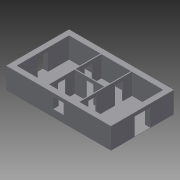
# Autodesk Inventor part: East_Structure
Saved by Autodesk Inventor 2013 SP2 (Build 170200200, 200)
## iProperties
Created: 2014-07-16
Part Number: East_Structure
Material: Generic
Document SubType Name: Modeling
Designer: jmw3
Density: 1 g/cm^3
Author: jmw3
Autodesk Inventor part; units mm, degrees
ref_plane "YZ Plane" through (0, 0, 0) normal (1, 0, 0) x (0, 1, 0)
ref_plane "XZ Plane" through (0, 0, 0) normal (0, 1, 0) x (-1, 0, 0)
ref_plane "XY Plane" through (0, 0, 0) normal (0, 0, 1) x (1, 0, 0)
sketch "Sketch1" plane through (0, 0, 0) normal (0, 1, 0) x (-1, 0, 0)
  line L0 (3657.6, -6096) -> (3657.6, 6096)
  line L1 (-3657.6, 6096) -> (-3657.6, -6096)
  line L2 (-5120.64, 0) -> (5120.64, 0) projected
  line L3 (0, -16303.5007) -> (0, 17151.3473) projected
  line L4 (-3048, 1714.5) -> (-3048, -1714.5)
  line L5 (3048, -5486.4) -> (3048, -1828.8)
  line L6 (3048, -1714.5) -> (3048, 1714.5)
  line L7 (3048, 1828.8) -> (3048, 5486.4)
  line L8 (-3048, -1828.8) -> (-3048, -5486.4)
  line L9 (-3048, 5486.4) -> (-3048, 1828.8)
  line L10 (-3048, 1714.5) -> (-3048, -1714.5)
  line L11 (-2009.775, -1828.8) -> (-2009.775, -1714.5)
  line L12 (-1095.375, -1828.8) -> (-1095.375, -1714.5)
  line L13 (-3048, -1714.5) -> (-2009.775, -1714.5)
  line L14 (-1095.375, -1714.5) -> (-57.15, -1714.5)
  line L15 (-3048, -1828.8) -> (-2009.775, -1828.8)
  line L16 (2009.775, -1828.8) -> (2009.775, -1714.5)
  line L17 (1095.375, -1828.8) -> (1095.375, -1714.5)
  line L18 (3048, -1714.5) -> (2009.775, -1714.5)
  line L19 (1095.375, -1714.5) -> (57.15, -1714.5)
  line L20 (3048, -1828.8) -> (2009.775, -1828.8)
  line L21 (1095.375, -1828.8) -> (-1095.375, -1828.8)
  line L22 (-2009.775, -1828.8) -> (-3048, -1828.8)
  line L23 (-1095.375, -1828.8) -> (1095.375, -1828.8)
  line L24 (2009.775, -1828.8) -> (3048, -1828.8)
  line L25 (57.15, -1714.5) -> (1095.375, -1714.5)
  line L26 (2009.775, -1714.5) -> (3048, -1714.5)
  line L27 (-2009.775, 1828.8) -> (-2009.775, 1714.5)
  line L28 (-1095.375, 1828.8) -> (-1095.375, 1714.5)
  line L29 (-3048, 1714.5) -> (-2009.775, 1714.5)
  line L30 (-1095.375, 1714.5) -> (-57.15, 1714.5)
  line L31 (-3048, 1828.8) -> (-2009.775, 1828.8)
  line L32 (3048, 1714.5) -> (2009.775, 1714.5)
  line L33 (3048, 1828.8) -> (2009.775, 1828.8)
  line L34 (2009.775, 1828.8) -> (2009.775, 1714.5)
  line L35 (1095.375, 1828.8) -> (1095.375, 1714.5)
  line L36 (1095.375, 1714.5) -> (57.15, 1714.5)
  line L37 (1095.375, 1828.8) -> (-1095.375, 1828.8)
  line L38 (-2009.775, 1828.8) -> (-3048, 1828.8)
  line L39 (-1095.375, 1828.8) -> (1095.375, 1828.8)
  line L40 (2009.775, 1828.8) -> (3048, 1828.8)
  line L41 (57.15, 1714.5) -> (1095.375, 1714.5)
  line L42 (2009.775, 1714.5) -> (3048, 1714.5)
  line L43 (-57.15, -457.2) -> (57.15, -457.2)
  line L44 (57.15, 457.2) -> (-57.15, 457.2)
  line L45 (-609.6, -6096) -> (-609.6, -5486.4)
  line L46 (609.6, -6096) -> (609.6, -5486.4)
  line L47 (-3048, -5486.4) -> (-609.6, -5486.4)
  line L48 (609.6, -5486.4) -> (3048, -5486.4)
  line L49 (-3657.6, -6096) -> (-609.6, -6096)
  line L50 (609.6, -6096) -> (3657.6, -6096)
  line L51 (914.4, 5486.4) -> (914.4, 6096)
  line L52 (-914.4, 6096) -> (-914.4, 5486.4)
  line L53 (3048, 5486.4) -> (914.4, 5486.4)
  line L54 (-914.4, 5486.4) -> (-3048, 5486.4)
  line L55 (3657.6, 6096) -> (914.4, 6096)
  line L56 (-914.4, 6096) -> (-3657.6, 6096)
  line L57 (-57.15, -1714.5) -> (-57.15, -457.2)
  line L58 (-57.15, 457.2) -> (-57.15, 1714.5)
  line L59 (-57.15, 1714.5) -> (-57.15, 457.2)
  line L60 (-57.15, -457.2) -> (-57.15, -1714.5)
  line L61 (57.15, -1714.5) -> (57.15, -457.2)
  line L62 (57.15, 457.2) -> (57.15, 1714.5)
  line L63 (57.15, 1714.5) -> (57.15, 457.2)
  line L64 (57.15, -457.2) -> (57.15, -1714.5)
  line L65 (-3048, 5486.4) -> (-3048, 1828.8)
  line L66 (-3048, 1828.8) -> (-2009.775, 1828.8)
  line L67 (-2009.775, 1828.8) -> (-2009.775, 1714.5)
  line L68 (-2009.775, 1714.5) -> (-3048, 1714.5)
  line L69 (-3048, 1714.5) -> (-3048, -1714.5)
  line L70 (-3048, -1714.5) -> (-2009.775, -1714.5)
  line L71 (-2009.775, -1714.5) -> (-2009.775, -1828.8)
  line L72 (-2009.775, -1828.8) -> (-3048, -1828.8)
  line L73 (-3048, -1828.8) -> (-3048, -5486.4)
  line L74 (-3048, -5486.4) -> (-609.6, -5486.4)
  line L75 (609.6, -5486.4) -> (3048, -5486.4)
  line L76 (3048, -5486.4) -> (3048, -1828.8)
  line L77 (3048, -1828.8) -> (2009.775, -1828.8)
  line L78 (2009.775, -1828.8) -> (2009.775, -1714.5)
  line L79 (2009.775, -1714.5) -> (3048, -1714.5)
  line L80 (3048, 1714.5) -> (3048, -1714.5)
  line L81 (3048, 1714.5) -> (2009.775, 1714.5)
  line L82 (2009.775, 1714.5) -> (2009.775, 1828.8)
  line L83 (2009.775, 1828.8) -> (3048, 1828.8)
  line L84 (3048, 1828.8) -> (3048, 5486.4)
  point P0 (0, 0)
  point P1 (0, 16303.5007)
  point P2 (0, -17151.3473)
  dimension "d2" = 7315.2
  dimension "d10" = 609.6
  dimension "d13" = 1038.225
  dimension "d14" = 914.4
  dimension "d17" = 114.3
  dimension "d18" = 1038.225
  dimension "d19" = 1038.225
  dimension "d20" = 914.4
  dimension "d21" = 1219.2
  dimension "d23" = 609.6
  dimension "d24" = 4267.2
  dimension "d25" = 1828.8
  dimension "d26" = 12192
  dimension "d27" = 609.6
  dimension "d28" = 114.3
  constraints: 166 end point, 46 perpendicular, 24 collinear, 24 symmetric about line, 23 parallel, 7 horizontal, 8 other
  measures "d2" distance between parallel lines of L0 L1
  measures "d10" distance between parallel lines of L0 L5
  measures "d13" distance between parallel lines of L10 L11
  measures "d14" distance between parallel lines of L11 L12
  measures "d17" distance between parallel lines of L23 L19
  measures "d18" distance of L4.start L29.end
  measures "d19" distance of L6.end L32.end
  measures "d20" distance between parallel lines of L43 L44
  measures "d21" distance between parallel lines of L46 L45
  measures "d23" distance between parallel lines of L49 L47
  measures "d24" distance between parallel lines of L15 L49
  measures "d25" distance between parallel lines of L51 L52
  measures "d26" distance between parallel lines of L50 L55
  measures "d27" distance between parallel lines of L56 L54
  measures "d28" distance between parallel lines of L64 L57
extrude "Extrusion1" add sketch "Sketch1" along normal blind 2438.4
sketch "Sketch2" plane through (-3657.6, 0, -6096) normal (-1, 0, 0) x (0, 0, 1)
  line L0 (0, 0) -> (12192, 0) projected
  line L1 (5486.4, 2032) -> (6705.6, 2032)
  line L2 (6705.6, 2032) -> (6705.6, 812.8)
  line L3 (6705.6, 812.8) -> (5486.4, 812.8)
  line L4 (5486.4, 812.8) -> (5486.4, 2032)
  line L5 (6096, 2926.08) -> (6096, -487.68) projected
  point P0 (6096, 0)
  dimension "d31" = 1219.2
  dimension "d33" = 1219.2
  dimension "d34" = 812.8
  constraints: 8 end point, 2 parallel, 1 horizontal, 1 perpendicular, 1 other
  measures "d31" distance between parallel lines of L2 L4
  measures "d33" distance between parallel lines of L1 L3
  measures "d34" distance between parallel lines of L0 L3
extrude "Extrusion2" cut sketch "Sketch2" against normal up to surface (609.6 mm away)
sketch "Sketch3" plane through (0, 2438.4, 0) normal (0, 1, 0) x (1, 0, 0)
  line L0 (57.15, 1714.5) -> (1095.375, 1714.5) projected
  line L1 (1095.375, 1714.5) -> (1095.375, 1828.8) projected
  line L2 (1095.375, 1828.8) -> (-1095.375, 1828.8) projected
  line L3 (-1095.375, 1828.8) -> (-1095.375, 1714.5) projected
  line L4 (-1095.375, 1714.5) -> (-57.15, 1714.5) projected
  line L5 (-57.15, 1714.5) -> (-57.15, 457.2) projected
  line L6 (-57.15, 457.2) -> (57.15, 457.2) projected
  line L7 (57.15, 457.2) -> (57.15, 1714.5) projected
  line L8 (-57.15, -1714.5) -> (-1095.375, -1714.5) projected
  line L9 (-1095.375, -1714.5) -> (-1095.375, -1828.8) projected
  line L10 (-1095.375, -1828.8) -> (1095.375, -1828.8) projected
  line L11 (1095.375, -1828.8) -> (1095.375, -1714.5) projected
  line L12 (1095.375, -1714.5) -> (57.15, -1714.5) projected
  line L13 (57.15, -1714.5) -> (57.15, -457.2) projected
  line L14 (57.15, -457.2) -> (-57.15, -457.2) projected
  line L15 (-57.15, -457.2) -> (-57.15, -1714.5) projected
  line L16 (3657.6, 6096) -> (609.6, 6096) projected
  line L17 (609.6, 6096) -> (609.6, 5486.4) projected
  line L18 (609.6, 5486.4) -> (3048, 5486.4) projected
  line L19 (3048, 5486.4) -> (3048, 1828.8) projected
  line L20 (3048, 1828.8) -> (2009.775, 1828.8) projected
  line L21 (2009.775, 1828.8) -> (2009.775, 1714.5) projected
  line L22 (2009.775, 1714.5) -> (3048, 1714.5) projected
  line L23 (3048, 1714.5) -> (3048, -1714.5) projected
  line L24 (3048, -1714.5) -> (2009.775, -1714.5) projected
  line L25 (2009.775, -1714.5) -> (2009.775, -1828.8) projected
  line L26 (2009.775, -1828.8) -> (3048, -1828.8) projected
  line L27 (3048, -1828.8) -> (3048, -5486.4) projected
  line L28 (3048, -5486.4) -> (914.4, -5486.4) projected
  line L29 (914.4, -5486.4) -> (914.4, -6096) projected
  line L30 (914.4, -6096) -> (3657.6, -6096) projected
  line L31 (3657.6, -6096) -> (3657.6, 6096) projected
  line L32 (-609.6, 6096) -> (609.6, 6096)
  line L33 (609.6, 6096) -> (609.6, 5486.4)
  line L34 (609.6, 5486.4) -> (-609.6, 5486.4)
  line L35 (-609.6, 5486.4) -> (-609.6, 6096)
  line L36 (-2009.775, 1828.8) -> (-1095.375, 1828.8)
  line L37 (-1095.375, 1828.8) -> (-1095.375, 1714.5)
  line L38 (-1095.375, 1714.5) -> (-2009.775, 1714.5)
  line L39 (-2009.775, 1714.5) -> (-2009.775, 1828.8)
  line L40 (1095.375, 1828.8) -> (2009.775, 1828.8)
  line L41 (2009.775, 1828.8) -> (2009.775, 1714.5)
  line L42 (2009.775, 1714.5) -> (1095.375, 1714.5)
  line L43 (1095.375, 1714.5) -> (1095.375, 1828.8)
  line L44 (-57.15, 457.2) -> (57.15, 457.2)
  line L45 (57.15, 457.2) -> (57.15, -457.2)
  line L46 (57.15, -457.2) -> (-57.15, -457.2)
  line L47 (-57.15, -457.2) -> (-57.15, 457.2)
  line L48 (1095.375, -1714.5) -> (2009.775, -1714.5)
  line L49 (2009.775, -1714.5) -> (2009.775, -1828.8)
  line L50 (2009.775, -1828.8) -> (1095.375, -1828.8)
  line L51 (1095.375, -1828.8) -> (1095.375, -1714.5)
  line L52 (-2009.775, -1714.5) -> (-1095.375, -1714.5)
  line L53 (-1095.375, -1714.5) -> (-1095.375, -1828.8)
  line L54 (-1095.375, -1828.8) -> (-2009.775, -1828.8)
  line L55 (-2009.775, -1828.8) -> (-2009.775, -1714.5)
  line L56 (-914.4, -5486.4) -> (914.4, -5486.4)
  line L57 (914.4, -5486.4) -> (914.4, -6096)
  line L58 (914.4, -6096) -> (-914.4, -6096)
  line L59 (-914.4, -6096) -> (-914.4, -5486.4)
  line L60 (1095.375, 1828.8) -> (2009.775, 1828.8)
  line L61 (2009.775, 1828.8) -> (2009.775, 1714.5)
  line L62 (2009.775, 1714.5) -> (1095.375, 1714.5)
  line L63 (1095.375, 1714.5) -> (1095.375, 1828.8)
  point P0 (0, 0)
  constraints: 64 end point, 16 parallel, 8 horizontal, 8 perpendicular
extrude "Extrusion3" add sketch "Sketch3" against normal blind 406.4 contours L1 L40 L21 L42 | L45 L14 L47 L6 | L3 L38 L39 L36 | L48 L25 L50 L11 | L9 L54 L55 L52 | L34 L35 L32 L17 | L29 L58 L59 L56
sketch "Sketch4" plane through (0, 2032, 0) normal (0, -1, 0) x (1, 0, 0)
  line L0 (914.4, 6096) -> (-914.4, 6096) projected
  line L1 (-914.4, 5486.4) -> (914.4, 5486.4) projected
  line L2 (0, 8534.4) -> (0, -8534.4) projected
  line L3 (-12.7, 6096) -> (12.7, 6096)
  line L4 (12.7, 6096) -> (12.7, 5486.4)
  line L5 (12.7, 5486.4) -> (-12.7, 5486.4)
  line L6 (-12.7, 5486.4) -> (-12.7, 6096)
  point P0 (0, 0)
  dimension "d39" = 25.4
  constraints: 8 end point, 2 parallel, 2 point on line, 1 horizontal, 1 perpendicular, 1 other
  measures "d39" distance between parallel lines of L4 L6
extrude "Extrusion4" add sketch "Sketch4" along normal blind 25.4
sketch "Sketch5" plane through (0, 0, 0) normal (0, -1, 0) x (1, 0, 0)
  line L0 (3657.6, -6096) -> (609.6, -6096) projected
  line L1 (3657.6, 6096) -> (3657.6, -6096) projected
  line L2 (914.4, 6096) -> (3657.6, 6096) projected
  line L3 (914.4, 5486.4) -> (914.4, 6096) projected
  line L4 (3048, 5486.4) -> (914.4, 5486.4) projected
  line L5 (3048, 1828.8) -> (3048, 5486.4) projected
  line L6 (2009.775, 1828.8) -> (3048, 1828.8) projected
  line L7 (2009.775, 1714.5) -> (2009.775, 1828.8) projected
  line L8 (3048, 1714.5) -> (2009.775, 1714.5) projected
  line L9 (3048, -1714.5) -> (3048, 1714.5) projected
  line L10 (2009.775, -1714.5) -> (3048, -1714.5) projected
  line L11 (2009.775, -1828.8) -> (2009.775, -1714.5) projected
  line L12 (3048, -1828.8) -> (2009.775, -1828.8) projected
  line L13 (3048, -5486.4) -> (3048, -1828.8) projected
  line L14 (609.6, -5486.4) -> (3048, -5486.4) projected
  line L15 (609.6, -6096) -> (609.6, -5486.4) projected
  line L16 (-3657.6, 6096) -> (3657.6, 6096)
  line L17 (3657.6, 6096) -> (3657.6, -6096)
  line L18 (3657.6, -6096) -> (-3657.6, -6096)
  line L19 (-3657.6, -6096) -> (-3657.6, 6096)
  point P0 (0, 0)
  constraints: 8 end point, 2 parallel, 1 horizontal, 1 perpendicular
extrude "Extrusion5" add sketch "Sketch5" along normal blind 25.4
body "Solid1"
